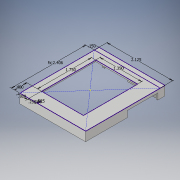
# Autodesk Inventor part: lisa
Saved by Autodesk Inventor 2017 (Build 210142000, 142)
## iProperties
Created: 2018-04-19
Part Number: lisa
Material: Generic
Document SubType Name: Modeling
Designer: Chad
Density: 1 g/cm^3
Appearance: Default
Author: Chad
Autodesk Inventor part; units mm, degrees
ref_plane "YZ Plane" through (0, 0, 0) normal (1, 0, 0) x (0, 1, 0)
ref_plane "XZ Plane" through (0, 0, 0) normal (0, 1, 0) x (-1, 0, 0)
ref_plane "XY Plane" through (0, 0, 0) normal (0, 0, 1) x (1, 0, 0)
sketch "Top Plate" plane through (0, 0, 0) normal (0, 1, 0) x (-1, 0, 0)
  line L0 (-26.9875, 30.5562) -> (26.9875, 30.5562)
  line L1 (26.9875, 30.5562) -> (26.9875, -30.5562)
  line L2 (26.9875, -30.5562) -> (-26.9875, -30.5562)
  line L3 (-26.9875, -30.5562) -> (-26.9875, 30.5562)
  line L4 (-26.9875, 30.5562) -> (26.9875, -30.5562) construction
  line L5 (26.9875, 30.5562) -> (-26.9875, -30.5562) construction
  line L6 (19.3675, 20.3962) -> (-14.9225, 20.3962)
  line L7 (-14.9225, 20.3962) -> (-14.9225, -24.0538)
  line L8 (-14.9225, -24.0538) -> (19.3675, -24.0538)
  line L9 (19.3675, -24.0538) -> (19.3675, 20.3962)
  line L10 (18.9103, 30.5562) -> (18.2753, 30.5562)
  line L11 (12.3825, 28.0162) -> (13.0175, 28.0162)
  line L12 (13.0175, 28.0162) -> (13.0175, 30.5562)
  line L13 (13.0175, 30.5562) -> (12.3825, 30.5562)
  line L14 (12.3825, 30.5562) -> (12.3825, 28.0162)
  line L15 (26.9875, -30.5562) -> (-26.9875, -30.5562)
  line L16 (-26.9875, -30.5562) -> (-26.9875, -34.3662)
  line L17 (-26.9875, -34.3662) -> (26.9875, -34.3662)
  line L18 (26.9875, -34.3662) -> (26.9875, -30.5562)
  point P0 (0, 0)
  dimension "d0" = 53.975
  dimension "d1" = 61.1124
  dimension "d7" = 44.45
  dimension "d8" = 34.29
  dimension "d9" = 7.62
  dimension "d10" = 10.16
  dimension "d48" = 0.635
  dimension "d49" = 6.35
  dimension "d50" = 2.54
  dimension "d77" = 3.81
  constraints: 38 end point, 8 parallel, 5 horizontal, 4 perpendicular, 2 midpoint, 2 point on line, 1 collinear
  measures "d0" distance of L1.end L2.end
  measures "d1" distance between parallel lines of L2 L0
  measures "d7" distance between parallel lines of L8 L6
  measures "d8" distance of L7.end L8.end
  measures "d9" distance from line of L1 L6.start
  measures "d10" vertical distance of L0.end L6.start
  measures "d48" distance of L11.start L11.end
  measures "d49" distance between parallel lines of L12 L9
  measures "d50" distance from line of L11 L12.end
  measures "d77" distance of L17.end L1.end
extrude "Top Plate Ext" add sketch "Top Plate" against normal blind 7.62 contours L0 L14 L11 L12 L1 L2 L3 | L0 L12 L11 L14 | L9 L8 L7 L6
shell "Top Plate Shell" thickness 1.27 removed faces 1 at (8.9958, -7.62, 10.1854)
extrude "Display Cutout" cut sketch "Top Plate" against normal blind 1.27 contours L9 L8 L7 L6
sketch "Power Btn" plane through (26.9875, 0, 30.5562) normal (1, 0, 0) x (0, 0, -1)
  line L0 (59.8424, -7.62) -> (1.27, -7.62) projected
  line L1 (59.2074, -7.62) -> (34.4424, -7.62)
  line L2 (34.4424, -7.62) -> (34.4424, -2.54)
  line L3 (34.4424, -2.54) -> (59.2074, -2.54)
  line L4 (59.2074, -2.54) -> (59.2074, -7.62)
  line L5 (61.1124, 0) -> (61.1124, -7.62) projected
  line L6 (61.1124, 0) -> (0, 0) projected
  point P0 (30.5562, 0)
  dimension "d18" = 1.905
  dimension "d19" = 24.765
  dimension "d20" = 2.54
  constraints: 8 end point, 2 parallel, 1 horizontal, 1 perpendicular, 1 point on line
  measures "d18" distance between parallel lines of L5 L4
  measures "d19" distance of L1.start L1.end
  measures "d20" distance between parallel lines of L6 L3
sketch "Dial/Vol" plane through (26.9875, 0, -30.5562) normal (0, 0, -1) x (-1, 0, 0)
  line L0 (53.975, -7.62) -> (0, -7.62) projected
  line L1 (52.705, -7.62) -> (46.355, -7.62)
  line L2 (46.355, -7.62) -> (46.355, -2.54)
  line L3 (46.355, -2.54) -> (52.705, -2.54)
  line L4 (52.705, -2.54) -> (52.705, -7.62)
  line L5 (53.975, 0) -> (0, 0) projected
  line L6 (52.705, -1.27) -> (52.705, -7.62) projected
  line L7 (1.27, -7.62) -> (52.705, -7.62) projected
  line L8 (44.323, -7.62) -> (25.273, -7.62)
  line L9 (25.273, -7.62) -> (25.273, -2.54)
  line L10 (25.273, -2.54) -> (44.323, -2.54)
  line L11 (44.323, -2.54) -> (44.323, -7.62)
  point P0 (26.9875, 0)
  dimension "d23" = 2.54
  dimension "d24" = 6.35
  dimension "d25" = 2.032
  dimension "d26" = 19.05
  constraints: 16 end point, 4 parallel, 2 collinear, 2 horizontal, 2 perpendicular, 2 point on line
  measures "d23" distance between parallel lines of L5 L3
  measures "d24" distance between parallel lines of L4 L2
  measures "d25" distance between parallel lines of L2 L11
  measures "d26" distance of L8.start L8.end
extrude "Power Cutout" cut sketch "Power Btn" against normal blind 1.27
extrude "Dial/Vol Cutout1" cut sketch "Dial/Vol" along normal blind 3.81 and the other way blind 1.27
sketch "SD Port" plane through (-26.9875, 0, -30.5562) normal (-1, 0, 0) x (0, 0, 1)
  line L0 (22.3774, -6.604) -> (46.5074, -6.604)
  line L1 (46.5074, -6.604) -> (46.5074, -2.794)
  line L2 (46.5074, -2.794) -> (22.3774, -2.794)
  line L3 (22.3774, -2.794) -> (22.3774, -6.604)
  line L4 (61.1124, 0) -> (0, 0) projected
  point P0 (30.5562, 0)
  point P1 (50.9524, 0)
  dimension "d31" = 2.794
  dimension "d32" = 3.81
  dimension "d33" = 24.13
  dimension "d34" = 4.445
  constraints: 8 end point, 2 parallel, 1 horizontal, 1 perpendicular
  measures "d31" distance between parallel lines of L4 L2
  measures "d32" distance of L0.end L1.end
  measures "d33" distance of L2.end L1.end
  measures "d34" distance from line of point (50.952, 0) L1
extrude "SD Port Cutout" cut sketch "SD Port" against normal blind 1.27
sketch "Display Pins" plane through (-25.7175, -1.27, -29.2862) normal (0, -1, 0) x (1, 0, 0)
  line L0 (40.64, 50.9524) -> (6.35, 50.9524)
  line L1 (6.35, 50.9524) -> (6.35, 53.4924)
  line L2 (6.35, 53.4924) -> (40.64, 53.4924)
  line L3 (40.64, 53.4924) -> (40.64, 50.9524)
  line L4 (40.64, 49.6824) -> (40.64, 5.2324) projected
  line L5 (6.35, 5.2324) -> (6.35, 49.6824) projected
  point P0 (25.7175, 29.2862)
  dimension "d56" = 1.27
  dimension "d57" = 2.54
  constraints: 8 end point, 2 collinear, 2 parallel, 1 horizontal, 1 perpendicular
  measures "d56" distance of L4.start L0.start
  measures "d57" distance of L2.end L0.start
extrude "Display Pins Cutout" cut sketch "Display Pins" against normal blind 1.016
extrude "M3 Screw Ext" add sketch "Top Plate" against normal blind 7.62 contours L2 L18 L17 L16
extrude "Dial/Vol Cutout2" cut sketch "Dial/Vol" along normal blind 7.62
body "Solid1"
